# Autodesk Inventor part: 0_005
Saved by Autodesk Inventor 2016 (Build 200138000, 138)
## iProperties
Created: 2016-04-08
Part Number: 0_005
Material: Generic
Document SubType Name: Modeling
Designer: Paschalis
Density: 1 g/cm^3
Appearance: LVK25, 0_005
Author: Paschalis
Autodesk Inventor part; units mm, degrees
ref_plane "YZ Plane" through (0, 0, 0) normal (1, 0, 0) x (0, 1, 0)
ref_plane "XZ Plane" through (0, 0, 0) normal (0, 1, 0) x (-1, 0, 0)
ref_plane "XY Plane" through (0, 0, 0) normal (0, 0, 1) x (1, 0, 0)
sketch "LVK25, 0_005_89" plane through (0, 0, 0) normal (0, 0, 1) x (1, 0, 0)
  line L0 (-1.6635, 3.2635) -> (1.6, 3.2635)
  line L1 (1.6, 3.2635) -> (1.6, -3.2635)
  line L2 (1.6, -3.2635) -> (-1.6635, -3.2635)
  line L3 (-1.6635, -3.2635) -> (-1.6635, 3.2635)
  constraints: 8 end point
extrude "Extrusion1" add sketch "LVK25, 0_005_89" along normal blind 1
body "Solid1"
